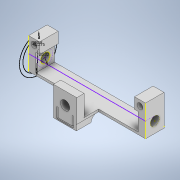
# Autodesk Inventor part: front 3-1
Saved by Autodesk Inventor 2020 (Build 240168000, 168)
## iProperties
Created: 2020-03-02
Part Number: front 3-1
Material: Generic
Document SubType Name: Modeling
Designer: akend
Density: 1 g/cm^3
Appearance: Default
Author: akend
Autodesk Inventor part; units mm, degrees
ref_plane "YZ Plane" through (0, 0, 0) normal (1, 0, 0) x (0, 1, 0)
ref_plane "XZ Plane" through (0, 0, 0) normal (0, 1, 0) x (-1, 0, 0)
ref_plane "XY Plane" through (0, 0, 0) normal (0, 0, 1) x (1, 0, 0)
sketch "Sketch1" plane through (0, 0, 0) normal (1, 0, 0) x (0, 1, 0)
  point P0 (0, 0)
sketch "Sketch2" plane through (0, 0, 0) normal (1, 0, 0) x (0, 1, 0)
  line L0 (0, 0) -> (25.4, 0)
  line L1 (25.4, 0) -> (25.4, 25.4)
  line L2 (25.4, 25.4) -> (0, 25.4)
  line L3 (0, 25.4) -> (0, 0)
  circle A0 centre (12.7, 12.7) radius 6.35
  dimension "d3" = 25.4
  dimension "d4" = 25.4
  dimension "d5" = 12.7
  constraints: 8 end point, 2 parallel, 1 centre point, 1 horizontal, 1 perpendicular
  measures "d3" distance of L2.end L1.end
  measures "d4" distance of L1.end L0.end
  measures "d5" diameter of A0
extrude "Extrusion1" add sketch "Sketch2" along normal blind 10
sketch "Sketch3" plane through (0, 0, 25.4) normal (0, 0, 1) x (1, 0, 0)
  line L0 (0, 0) -> (0, 25.4) projected
  line L1 (0, 25.4) -> (15, 25.4)
  line L2 (15, 25.4) -> (15, 40.4)
  line L3 (15, 40.4) -> (0, 40.4)
  line L4 (0, 40.4) -> (0, 25.4)
  circle A0 centre (7.5, 32.9) radius 4
  dimension "d8" = 15
  dimension "d9" = 15
  dimension "d10" = 8
  constraints: 8 end point, 2 parallel, 1 centre point, 1 horizontal, 1 perpendicular
  measures "d8" distance of L3.end L2.end
  measures "d9" distance of L2.end L1.end
  measures "d10" diameter of A0
extrude "Extrusion2" add sketch "Sketch3" against normal blind 25.4
sketch "Sketch4" plane through (0, 40.4, 25.4) normal (0, 1, 0) x (1, 0, 0)
  line L0 (15, 25.4) -> (10, 25.4) projected
  line L1 (15, 19.05) -> (15, 25.4)
  line L2 (15, 25.4) -> (0, 25.4)
  line L3 (0, 25.4) -> (0, 19.05)
  line L4 (15, 19.05) -> (0, 19.05)
  line L5 (15, 0) -> (15, 25.4) projected
  point P0 (0, 0)
  constraints: 8 end point, 1 parallel, 1 perpendicular
extrude "Extrusion3" add sketch "Sketch4" against normal blind 14.85
sketch "Sketch5" plane through (10, 0, 0) normal (1, 0, 0) x (0, 0, -1)
  circle A0 centre (-12.7, 12.7) radius 10.16 construction
  point P0 (0, 0)
  dimension "d16" = 20.32
  constraints: 1 centre point, 1 coincident
  measures "d16" diameter of A0
sketch "Sketch6" plane through (0, 0, 0) normal (-1, 0, 0) x (0, 0, 1)
  circle A0 centre (12.7, 12.7) radius 6.35 projected
  circle A1 centre (12.7, 12.7) radius 20.6375
  point P0 (0, 0)
  dimension "d17" = 41.275
  constraints: 1 centre point, 1 coincident
  measures "d17" diameter of A1
sketch "Sketch7" plane through (10, 0, 0) normal (1, 0, 0) x (0, 0, -1)
  line L0 (0, 0) -> (0, -2)
  line L1 (0, -2) -> (-25.4, -2)
  line L2 (-25.4, -2) -> (-25.4, 0)
  line L3 (-25.4, 25.4) -> (-25.4, 0) projected
  line L4 (0, -2) -> (-25.4, -2)
  line L5 (-25.4, -2) -> (-25.4, 1.25)
  line L6 (-25.4, 1.25) -> (0, 1.25)
  line L7 (0, 1.25) -> (0, -2)
  dimension "d18" = 2
  dimension "d19" = 3.25
  constraints: 14 end point, 3 parallel, 1 horizontal, 1 perpendicular, 1 point on line
  measures "d18" distance of L0.start L0.end
  measures "d19" distance of L4.end L5.end
extrude "Extrusion4" add sketch "Sketch7" along normal blind 150 and the other way blind 10
sketch "Sketch8" plane through (10, 0, 0) normal (1, 0, 0) x (0, 0, -1)
  point P0 (0, 0)
sketch "Sketch9" plane through (160, 0, 0) normal (1, 0, 0) x (0, 0, -1)
  line L0 (-25.4, 25.4) -> (-25.4, 1.25) projected
  line L1 (-25.4, -2) -> (0, -2) projected
  line L2 (-25.4, 25.4) -> (0, 25.4)
  line L3 (0, 25.4) -> (0, -2)
  line L4 (0, -2) -> (-25.4, -2)
  line L5 (-25.4, -2) -> (-25.4, 25.4)
  circle A0 centre (-12.7, 12.7) radius 6.35 projected
  circle A1 centre (-12.7, 12.7) radius 6.35
  point P0 (0, 0)
  constraints: 8 end point, 2 parallel, 1 centre point, 1 coincident, 1 horizontal, 1 perpendicular
extrude "Extrusion5" add sketch "Sketch9" against normal blind 10
sketch "Sketch10" plane through (0, 40.4, 25.4) normal (0, 0, 1) x (1, 0, 0)
  line L0 (160, -15) -> (150, -15) projected
  line L1 (160, -15) -> (145, -15)
  line L2 (145, -15) -> (145, 0)
  line L3 (145, 0) -> (160, 0)
  line L4 (160, 0) -> (160, -15)
  circle A0 centre (152.5, -7.5) radius 4
  point P0 (0, -40.4)
  dimension "d26" = 15
  dimension "d27" = 15
  dimension "d28" = 8
  constraints: 8 end point, 2 parallel, 1 centre point, 1 horizontal, 1 perpendicular
  measures "d26" distance of L2.end L3.end
  measures "d27" distance of L1.end L2.end
  measures "d28" diameter of A0
extrude "Extrusion6" add sketch "Sketch10" against normal blind 25.4
sketch "Sketch11" plane through (0, 40.4, 25.4) normal (0, 1, 0) x (1, 0, 0)
  line L0 (0, 0) -> (160, 0) construction
  line L1 (15, 0) -> (15, 25.4) construction
  line L2 (0, 0) -> (15, 0) construction
  line L3 (15, 0) -> (15, 18) construction
  line L4 (15, 18) -> (0, 18) construction
  line L5 (0, 18) -> (0, 0) construction
  line L6 (0, 18) -> (15, 18)
  line L7 (15, 18) -> (15, 25.4)
  line L8 (15, 25.4) -> (0, 25.4)
  line L9 (0, 25.4) -> (0, 18)
  dimension "d31" = 18
  constraints: 16 end point, 4 parallel, 2 horizontal, 2 perpendicular, 1 point on line
  measures "d31" distance of L3.end L2.end
sketch "Sketch12" plane through (0, 40.4, 25.4) normal (0, 0, 1) x (1, 0, 0)
  circle A0 centre (7.5, -7.5) radius 4 projected
  circle A1 centre (7.5, -7.5) radius 4
  point P0 (0, -40.4)
  constraints: 1 centre point, 1 coincident
extrude "Extrusion7" cut sketch "Sketch12" against normal blind 25.4
sketch "Sketch13" plane through (145, 40.4, 25.4) normal (0, 1, 0) x (1, 0, 0)
  line L0 (0, 0) -> (0, 25.4) projected
  line L1 (15, 25.4) -> (0, 25.4)
  line L2 (0, 25.4) -> (0, 18)
  line L3 (0, 18) -> (15, 18)
  line L4 (15, 18) -> (15, 25.4)
  point P0 (-145, 25.4)
  dimension "d34" = 7.4
  constraints: 8 end point, 2 parallel, 1 horizontal, 1 perpendicular, 1 point on line
  measures "d34" distance of L2.end L1.end
extrude "Extrusion8" add sketch "Sketch13" against normal blind 14.9
extrude "Extrusion9" add sketch "Sketch11" against normal blind 14.9
sketch "Sketch14" plane through (0, 40.4, 25.4) normal (0, 0, 1) x (1, 0, 0)
  point P0 (0, -40.4)
sketch "Sketch15" plane through (10, 0, 0) normal (1, 0, 0) x (0, 0, -1)
  circle A0 centre (-12.7, 12.7) radius 6.35 projected
  point P0 (0, 0)
  constraints: 1 coincident
sketch "Sketch16" plane through (150, 0, 0) normal (-1, 0, 0) x (0, 0, 1)
  circle A0 centre (12.7, 12.7) radius 6.35 projected
  point P0 (0, 0)
  constraints: 1 coincident
sketch "Sketch17" plane through (0, 40.4, 25.4) normal (0, 0, 1) x (1, 0, 0)
  line L0 (10, -39.15) -> (10, -15) construction
  line L1 (10, -27.075) -> (150, -27.075) construction
  line L2 (150, -15) -> (150, -39.15) construction
  line L3 (10, -39.15) -> (150, -39.15) construction
  line L4 (80, -39.15) -> (80, -27.075) construction
  line L5 (95.875, -42.4) -> (64.125, -42.4)
  line L6 (64.125, -42.4) -> (64.125, -39.15)
  line L7 (64.125, -39.15) -> (95.875, -39.15)
  line L8 (95.875, -39.15) -> (95.875, -42.4)
  point P0 (0, -40.4)
  point P1 (80, -40.775)
  dimension "d39" = 31.75
  constraints: 12 end point, 4 midpoint, 2 parallel, 1 horizontal, 1 perpendicular, 1 point on line
  measures "d39" distance of L6.end L7.end
extrude "Extrusion10" add sketch "Sketch17" along normal blind 20
sketch "Sketch18" plane through (0, 40.4, 45.4) normal (0, 0, 1) x (1, 0, 0)
  line L0 (0, -42.4) -> (64.125, -42.4) projected
  line L1 (64.125, -42.4) -> (95.875, -42.4)
  line L2 (95.875, -42.4) -> (95.875, -17.4)
  line L3 (95.875, -17.4) -> (64.125, -17.4)
  line L4 (64.125, -17.4) -> (64.125, -42.4)
  point P0 (0, -40.4)
  dimension "d42" = 25
  constraints: 8 end point, 2 parallel, 1 horizontal, 1 perpendicular
  measures "d42" distance of L2.end L1.end
extrude "Extrusion11" add sketch "Sketch18" along normal blind 10
sketch "Sketch19" plane through (160, 0, 0) normal (1, 0, 0) x (0, 0, -1)
  circle A0 centre (-12.7, 12.7) radius 6.35 construction
  line L0 (-12.7, 19.05) -> (-25.4, 19.05) construction
  line L1 (-25.4, 40.4) -> (-25.4, -2) construction
  point P0 (0, 0)
  constraints: 2 end point, 1 horizontal, 1 point on line, 1 vertical alignment, 1 other
sketch "Sketch20" plane through (145, 40.4, 25.4) normal (0, 0, 1) x (1, 0, 0)
  line L0 (15, 0) -> (15, -42.4) projected
  line L1 (15, -21.35) -> (-145, -21.35)
  line L2 (-145, 0) -> (-145, -42.4) projected
  point P0 (-145, -40.4)
  constraints: 2 end point, 2 point on line, 1 horizontal
sketch "Sketch21" plane through (0, 40.4, 55.4) normal (0, 0, 1) x (1, 0, 0)
  line L0 (95.875, -39.15) -> (95.875, -42.4) projected
  line L1 (95.875, -42.4) -> (64.125, -42.4)
  line L2 (64.125, -42.4) -> (64.125, -10.65)
  line L3 (64.125, -10.65) -> (95.875, -10.65)
  line L4 (95.875, -10.65) -> (95.875, -42.4)
  point P0 (0, -40.4)
  dimension "d45" = 31.75
  constraints: 8 end point, 2 parallel, 1 horizontal, 1 perpendicular
  measures "d45" distance of L1.end L2.end
extrude "Extrusion12" add sketch "Sketch21" against normal blind 10
sketch "Sketch22" plane through (0, 40.4, 55.4) normal (0, 0, 1) x (1, 0, 0)
  circle A0 centre (80, -27.7) radius 6.35
  point P0 (0, -40.4)
  point P1 (80, -21.35)
  dimension "d48" = 12.7
  constraints: 1 centre point, 1 coincident
  measures "d48" diameter of A0
extrude "Extrusion13" cut sketch "Sketch22" against normal blind 10
sketch "Sketch23" plane through (0, 40.4, 55.4) normal (0, 0, 1) x (1, 0, 0)
  line L0 (64.125, -10.65) -> (64.125, -39.15) construction
  line L1 (64.125, -27.7833) -> (95.875, -27.7833) construction
  line L2 (95.875, -27.7833) -> (95.875, -48.7833) construction
  circle A0 centre (80, -27.7) radius 6.35 construction
  line L3 (95.875, -48.7833) -> (64.125, -48.7833) construction
  line L4 (91.25, -27.7833) -> (91.25, -48.7833) construction
  line L5 (68.75, -48.7833) -> (91.25, -48.7833) construction
  line L6 (91.25, -48.7833) -> (91.25, -47.1958) construction
  line L7 (91.25, -47.1958) -> (68.75, -47.1958) construction
  line L8 (68.75, -47.1958) -> (68.75, -48.7833) construction
  line L9 (91.25, -48.7833) -> (89.6625, -48.7833) construction
  line L10 (89.6625, -48.7833) -> (89.6625, -34.7833) construction
  line L11 (89.6625, -34.7833) -> (91.25, -34.7833) construction
  line L12 (91.25, -34.7833) -> (91.25, -48.7833) construction
  line L13 (68.75, -48.7833) -> (70.3375, -48.7833) construction
  line L14 (70.3375, -48.7833) -> (70.3375, -34.7833) construction
  line L15 (70.3375, -34.7833) -> (68.75, -34.7833) construction
  line L16 (68.75, -34.7833) -> (68.75, -48.7833) construction
  circle A1 centre (80, -27.7) radius 3.175 construction
  line L17 (80, -30.875) -> (95.875, -30.875) construction
  line L18 (95.875, -39.15) -> (95.875, -10.65) construction
  line L19 (68.75, -34.7833) -> (70.3375, -34.7833)
  line L20 (70.3375, -34.7833) -> (70.3375, -47.1958)
  line L21 (89.6625, -47.1958) -> (70.3375, -47.1958)
  line L22 (89.6625, -34.7833) -> (89.6625, -47.1958)
  line L23 (89.6625, -34.7833) -> (91.25, -34.7833)
  line L24 (91.25, -34.7833) -> (91.25, -48.7833)
  line L25 (91.25, -48.7833) -> (68.75, -48.7833)
  line L26 (68.75, -48.7833) -> (68.75, -34.7833)
  point P0 (0, -40.4)
  dimension "d61" = 6.35
  dimension "d51" = 21
  dimension "d58" = 1.5875
  dimension "d59" = 1.5875
  dimension "d60" = 1.5875
  constraints: 50 end point, 9 point on line, 7 perpendicular, 6 horizontal, 6 parallel, 5 collinear, 1 coincident, 1 vertical alignment, 2 other
  measures "d51" distance of L1.end L2.end
  measures "d58" distance of L6.end L5.end
  measures "d59" distance of L10.end L11.end
  measures "d60" distance of L15.end L14.end
sketch "Sketch24" plane through (0, 0, 0) normal (-1, 0, 0) x (0, 0, 1)
  circle A0 centre (12.7, 12.7) radius 6.35 projected
  circle A1 centre (12.7, 12.7) radius 25.4
  point P0 (0, 0)
  dimension "d62" = 50.8
  constraints: 1 centre point, 1 coincident
  measures "d62" diameter of A1
sketch "Sketch25" plane through (0, 40.4, 55.4) normal (0, 0, 1) x (1, 0, 0)
  line L0 (0, -42.4) -> (64.125, -42.4) projected
  line L1 (64.125, -42.4) -> (95.373, -42.4)
  line L2 (95.373, -42.4) -> (95.373, -50.4)
  line L3 (95.373, -50.4) -> (64.125, -50.4)
  line L4 (64.125, -50.4) -> (64.125, -42.4)
  point P0 (0, -40.4)
  dimension "d63" = 8
  constraints: 8 end point, 2 parallel, 1 horizontal, 1 perpendicular
  measures "d63" distance of L1.end L2.end
extrude "Extrusion14" add sketch "Sketch25" against normal blind 20
extrude "Extrusion15" cut sketch "Sketch23" against normal blind 15
fillet "Fillet1" radius 9 1 edges at (79.749, -2, 35.4)
body "Solid1"
